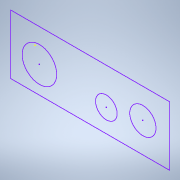
# Autodesk Inventor part: FahenVerbindung_maybe
Saved by Autodesk Inventor 2020.3 (Build 243373010, 373A)
## iProperties
Created: 2020-11-08
Part Number: FahenVerbindung_maybe
Material: Generisch
Document SubType Name: Modeling
Designer: Stefan
Density: 1 g/cm^3
Appearance: Vorgabe
Author: Stefan
Autodesk Inventor part; units mm, degrees
ref_plane "YZ Plane" through (0, 0, 0) normal (1, 0, 0) x (0, 1, 0)
ref_plane "XZ Plane" through (0, 0, 0) normal (0, 1, 0) x (-1, 0, 0)
ref_plane "XY Plane" through (0, 0, 0) normal (0, 0, 1) x (1, 0, 0)
sketch "Skizze1" plane through (0, 0, 0) normal (0, 0, 1) x (1, 0, 0)
  line L0 (-21.1699, -53.0641) -> (378.8301, -53.0641)
  line L1 (378.8301, -53.0641) -> (378.8301, -103.0641)
  line L2 (378.8301, -103.0641) -> (-21.1699, -103.0641)
  line L3 (-21.1699, -103.0641) -> (-21.1699, -53.0641)
  circle A0 centre (28.8301, -78.0641) radius 10
  circle A1 centre (178.8301, -78.0641) radius 10
  circle A2 centre (328.8301, -78.0641) radius 10
  point P0 (0, 0)
  dimension "d0" = 400
  dimension "d1" = 50
  dimension "d2" = 20
  dimension "d3" = 20
  dimension "d4" = 20
  dimension "d5" = 25
  dimension "d6" = 25
  dimension "d7" = 25
  dimension "d8" = 200
  dimension "d9" = 150
  dimension "d10" = 150
  constraints: 8 end point, 3 centre point, 2 parallel, 1 horizontal, 1 perpendicular
  measures "d0" distance of L1.end L2.end
  measures "d1" distance of L2.end L0.start
  measures "d2" diameter of A0
  measures "d3" diameter of A1
  measures "d4" diameter of A2
  measures "d5" distance from line of L2 A0.centre
  measures "d6" distance from line of L2 A1.centre
  measures "d7" distance from line of L2 A2.centre
  measures "d8" distance from line of L1 A1.centre
  measures "d9" distance of A2.centre A1.centre
  measures "d10" distance of A0.centre A1.centre
extrude "Extrusion1" add sketch "Skizze1" along normal blind 10
